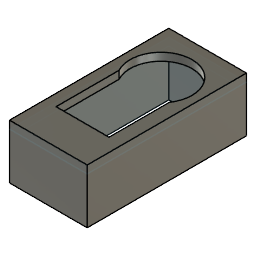
Servo enclosure (Autodesk Fusion 360 design; units mm, degrees)
Autodesk Fusion 360 part; units mm, degrees
sketch "Sketch1" plane through (0, 0, 0) normal (0, 0, 1) x (1, 0, 0)
  line L0 (0, 0) -> (12, 0)
  line L1 (12, 0) -> (12, 33)
  line L2 (12, 33) -> (0, 33)
  line L3 (0, 33) -> (0, 0)
  line L4 (-2, 35) -> (14, 35)
  line L5 (14, 35) -> (14, -2)
  line L6 (14, -2) -> (-2, -2)
  line L7 (-2, -2) -> (-2, 35)
  dimension "d1" = 33
  dimension "d2" = 12
  dimension "d3" = 2
  dimension "d4" = 2
  dimension "d5" = 2
  dimension "d6" = 2
  constraint horizontal L0
  constraint vertical L1
  constraint horizontal L2
  constraint vertical L3
  constraint coincident L0.start L3.end
  constraint horizontal L4
  constraint vertical L5
  constraint horizontal L6
  constraint vertical L7
  measures "d1" distance of L0.start L2.end
  measures "d2" distance of L0.start L0.end
  measures "d3" distance of L3 L7
  measures "d4" distance of L2 L4
  measures "d5" distance of L1 L5
  measures "d6" distance of L0 L6
extrude "Extrude1" add sketch "Sketch1" along normal blind 20 makes body 1
extrude "Extrude2" add sketch "Sketch1" against normal blind 2 contours L0 L1 L2 L3 | L4 L5 L6 L7 bodies 1
sketch "Sketch2" plane through (0, 0, 20) normal (0, 0, 1) x (-1, 0, 0)
  line L0 (0, 0) -> (0, -33)
  line L1 (0, -33) -> (-12, -33)
  line L2 (-12, -33) -> (-12, 0)
  line L3 (-12, 0) -> (0, 0)
  line L4 (2, 2) -> (-14, 2)
  line L5 (-14, 2) -> (-14, -35)
  line L6 (-14, -35) -> (2, -35)
  line L7 (2, -35) -> (2, 2)
  line L8 (4, 4) -> (-16, 4)
  line L9 (-16, 4) -> (-16, -37)
  line L10 (-16, -37) -> (4, -37)
  line L11 (4, -37) -> (4, 4)
  dimension "d11" = 2
extrude "Extrude3" add sketch "Sketch2" against normal blind 12 separate body contours L8 L9 L10 L11 makes body 2
sketch "Sketch3" plane through (0, 0, 20) normal (0, 0, 1) x (-1, 0, 0)
  line L0 (2, 2) -> (2, -35)
  line L1 (2, -35) -> (-14, -35)
  line L2 (-14, -35) -> (-14, 2)
  line L3 (-14, 2) -> (2, 2)
  line L4 (4, -37) -> (4, 4)
  line L5 (4, 4) -> (-16, 4)
  line L6 (-16, 4) -> (-16, -37)
  line L7 (-16, -37) -> (4, -37)
extrude "Extrude5" add sketch "Sketch3" along normal blind 2 contours L0 L1 L2 L3 | L4 L5 L6 L7 bodies 2
sketch "Sketch4" plane through (0, 0, 22) normal (0, 0, 1) x (-1, 0, 0)
  line L0 (-16, -37) -> (4, -37)
  line L1 (4, -37) -> (4, 4)
  line L2 (4, 4) -> (-16, 4)
  line L3 (-16, 4) -> (-16, -37)
  circle A0 centre (-6, -25) radius 7.9669
  line L4 (-12.5894, -20.5221) -> (-12.5894, -5)
  line L5 (-12.5894, -5) -> (1, -5)
  line L6 (1, -5) -> (1, -21.1958)
  dimension "d20" = 15.9338
  constraint coincident A0 L4.start
  constraint parallel L3 L4
  constraint perpendicular L4 L5
  constraint coincident A0 L6.end
  constraint perpendicular L5 L6
  measures "d20" diameter of A0
extrude "Extrude6" cut sketch "Sketch4" against normal blind 2 contours A0 | A0 L4 L5 L6 bodies 2
hidden bodies 1
